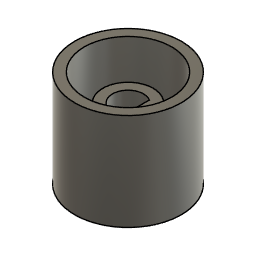
Knob (22mm) (Autodesk Fusion 360 design; units mm, degrees)
Autodesk Fusion 360 part; units mm, degrees
sketch "Outer" plane through (0, 0, 0) normal (0, 1, 0) x (1, 0, 0)
  circle A0 centre (0, 0) radius 11
  dimension "d1" = 22
  constraint coincident A0.centre origin
  measures "d1" diameter of A0
extrude "Extrude1" add sketch "Outer" along normal blind 20
sketch "Inner" plane through (0, 20, 0) normal (0, 1, 0) x (-1, 0, 0)
  circle A0 centre (0, 0) radius 11
  circle A1 centre (0, 0) radius 9
  dimension "d4" = 18
  constraint coincident A0.centre A1.centre
  measures "d4" diameter of A1
extrude "Extrude2" cut sketch "Inner" against normal blind 18 contours A1
sketch "Shaft" plane through (0, 2, 0) normal (0, 1, 0) x (-1, 0, 0)
  circle A0 centre (0, 0) radius 9
  line L0 (-1.7, 2.7111) -> (-1.7, -2.7111)
  arc A1 (-1.7, -2.7111) -> (-1.7, 2.7111) centre (0, 0) ccw
  arc A2 (-3.7, -3.6538) -> (-3.7, 3.6538) centre (0, 0) ccw
  line L1 (-3.7, 3.6538) -> (-3.7, -3.6538)
  dimension "d7" = 6.4
  dimension "d8" = 1.7
  dimension "d9" = 2
  constraint concentric A0 A1
  constraint vertical L0
  measures "d7" diameter of A1
  measures "d8" distance of A0.centre L0
extrude "Extrude3" add sketch "Shaft" along normal blind 12.5 contours A2 L1
extrude "Extrude4" add 1 faces at (0.0662, 2, 0.598) along direction (0, 1, 0) blind 5
equation "d5 = -( 20 mm - 2 mm )"
equation "d7 = 6 mm + 0.2 mm + 0.2 mm"
equation "d8 = ( 4.5 mm - 3 mm ) + 0.2 mm"
equation "d10 = 20 mm - 2 mm - 5.5 mm"
equation "d12 = 20 mm - 2 mm - 5.5 mm - 7.5 mm"
named bodies: "Body"
